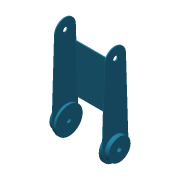
# Autodesk Inventor part: 2nd_Arm
Saved by Autodesk Inventor 2016 (Build 200138000, 138)
## iProperties
Created: 2015-05-19
Part Number: 2nd_Arm
Material: Aluminum 6061
Document SubType Name: Modeling
Designer: CHUNGBK
Density: 2.7 g/cm^3
Appearance: Turquoise
Mass: 770.248 g
Surface Area: 1350.92 cm^2
Volume: 285.277 cm^3
Author: CHUNGBK
Autodesk Inventor part; units mm, degrees
sketch "Sketch1" plane through (0, 0, 0) normal (1, 0, 0) x (0, 1, 0)
  circle A0 centre (0, 0) radius 31.75
  dimension "d0" = 63.5
  constraints: 1 centre point, 1 coincident
  measures "d0" diameter of A0
extrude "Extrusion1" add sketch "Sketch1" along normal blind 11.43
sketch "Sketch2" plane through (11.43, 0, 0) normal (1, 0, 0) x (0, 0, -1)
  circle A0 centre (0, 0) radius 36.83
  circle A1 centre (0, 0) radius 31.75 projected
  circle A2 centre (0, 220.6625) radius 29.845
  line L0 (-29.83, 221.6072) -> (-36.8115, 1.1658)
  line L1 (36.8115, 1.1658) -> (29.83, 221.6072)
  line L2 (0, 220.6625) -> (0, 0) construction
  dimension "d3" = 5.08
  dimension "d4" = 59.69
  dimension "d5" = 220.6625
  constraints: 6 end point, 4 point on circle, 4 tangent, 2 centre point, 1 coincident, 1 vertical
  measures "d3" radial gap between concentric circles of A0 A1
  measures "d4" diameter of A2
  measures "d5" distance of L2.start L2.end
extrude "Extrusion2" add sketch "Sketch2" along normal blind 2.794 contours A0 | A0 L0 A2 L1 | A2 | A1
ref_plane "Work Plane1" through (18.288, 0, 0) normal (1, 0, 0) x (0, 0, -1)
sketch "Sketch4" plane through (18.288, 0, 0) normal (1, 0, 0) x (0, 0, -1)
  circle A0 centre (0, 0) radius 39.116
  dimension "d12" = 78.232
  constraints: 1 centre point, 1 coincident
  measures "d12" diameter of A0
extrude "Extrusion4" add sketch "Sketch4" along normal blind 6.35
ref_plane "Work Plane2" through (155.5115, 0, 0) normal (1, 0, 0) x (0, 0, -1)
sketch "Sketch5" plane through (14.224, 0, 0) normal (1, 0, 0) x (0, 0, -1)
  line L0 (36.8115, 1.1658) -> (29.83, 221.6072) projected
  line L1 (35.6418, 38.1) -> (32.8492, 38.0116)
  line L2 (32.8492, 38.0116) -> (28.3768, 179.2283)
  line L3 (28.3768, 179.2283) -> (31.1694, 179.3167)
  point P0 (0, 0)
  dimension "d16" = 2.794
  dimension "d17" = 141.2875
  dimension "d18" = 38.1
  constraints: 6 end point, 2 perpendicular, 2 point on line, 1 parallel
  measures "d16" distance between parallel lines of L0 L2
  measures "d17" distance of L1.end L2.end
  measures "d18" vertical distance of point (0, 0) L1.start
extrude "Extrusion5" add sketch "Sketch5" along normal up to surface (141.2875 mm away)
ref_plane "Work Plane3" through (84.8678, 0, 0) normal (1, 0, 0) x (0, 0, -1)
mirror "Mirror1" about plane through (84.8678, 0, 0) normal (1, 0, 0) of "Extrusion2", "Extrusion1"
sketch "Sketch6" plane through (155.5115, 0, 0) normal (-1, 0, 0) x (0, 0, 1)
  circle A0 centre (0, 0) radius 39.116 projected
extrude "Extrusion6" add sketch "Sketch6" along normal blind 6.35
sketch "Sketch3" plane through (14.224, 0, 0) normal (1, 0, 0) x (0, 0, -1)
  circle A0 centre (0, 0) radius 6.35
  dimension "d8" = 12.7
  constraints: 1 centre point, 1 coincident
  measures "d8" diameter of A0
extrude "Extrusion3" cut sketch "Sketch3" along normal through all both and the other way through all
sketch "Sketch7" plane through (158.3055, 0, 0) normal (1, 0, 0) x (0, 0, -1)
  arc A0 (29.83, 221.6072) -> (-29.83, 221.6072) centre (0, 220.6625) ccw projected
  circle A1 centre (0, 220.6625) radius 6.35
  point P0 (0, 0)
  dimension "d24" = 12.7
  constraints: 1 centre point, 1 coincident
  measures "d24" diameter of A1
extrude "Extrusion7" cut sketch "Sketch7" against normal through all
body "Solid1"
